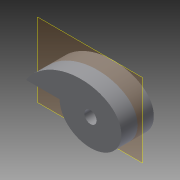
# Autodesk Inventor part: cam 1
Saved by Autodesk Inventor 2014 (Build 180170000, 170)
## iProperties
Created: 2014-05-19
Part Number: cam 1
Material: Generic
Document SubType Name: Modeling
Designer: jyesowitz
Density: 1 g/cm^3
Appearance: Default
Author: jyesowitz
Autodesk Inventor part; units mm, degrees
ref_plane "YZ Plane" through (0, 0, 0) normal (1, 0, 0) x (0, 1, 0)
ref_plane "XZ Plane" through (0, 0, 0) normal (0, 1, 0) x (-1, 0, 0)
ref_plane "XY Plane" through (0, 0, 0) normal (0, 0, 1) x (1, 0, 0)
sketch "Sketch1" plane through (0, 0, 0) normal (0, 0, 1) x (1, 0, 0)
  ellipse E0 centre (0.0254, -0.0123) end of major axis (24.1554, -0.0123) minor radius 20.8653 (-24.1046, -0.0123) -> (23.1482, 5.9531) ccw
  line L0 (23.1482, 5.9531) -> (16.5031, 25.2125) construction
  line L1 (16.5031, 25.2125) -> (-22.7223, 31.8008) construction
  line L2 (-22.7223, 31.8008) -> (-44.5279, 10.0148) construction
  line L3 (-44.5279, 10.0148) -> (-50.2984, -0.0123) construction
  spline S0 degree 4 poles (23.1482, 5.9531) (16.5031, 25.2125) (-22.7223, 31.8008) (-44.5279, 10.0148) (-50.2984, -0.0123) knots 1 1 1 1 1 2 2 2 2 2
  line L4 (-50.2984, -0.0123) -> (-24.1046, -0.0123)
  circle A0 centre (0.0254, -0.0123) radius 4.7625
  point P0 (0, 0)
  dimension "d62" = 24.13
  dimension "d63" = 20.8653
  dimension "d42" = 31.8008
  dimension "d43" = 50.2983
  dimension "d44" = 24.1046
  dimension "d45" = 30.8239
  dimension "d46" = 11.569
  dimension "d47" = 39.7748
  dimension "d48" = 20.3735
  dimension "d53" = 125.491
  dimension "d57" = 5.9531
  dimension "d64" = 9.525
  constraints: 2 end point, 1 centre point, 1 coincident, 1 horizontal, 1 horizontal alignment, 10 other
  measures "d42" vertical distance of point (0, 0) L1.end
  measures "d43" distance of point (0, 0) L3.end
  measures "d44" distance of point (0, 0) L4.end
  measures "d45" distance of L1.end L2.end
  measures "d46" distance of L2.end L3.end
  measures "d47" distance of L0.end L1.end
  measures "d48" distance of L0.start L0.end
  measures "d53" angle of L2 L1
  measures "d57" vertical distance of point (0, 0) L0.start
  measures "d64" diameter of A0
extrude "Extrusion1" add sketch "Sketch1" against normal blind 25.4
body "Solid1"
